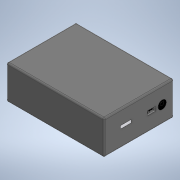
# Autodesk Inventor part: 22Ah BatteryPack
Saved by Autodesk Inventor 2021 (Build 250183000, 183)
## iProperties
Created: 2019-10-24
Part Number: 22Ah BatteryPack
Material: Generic
Document SubType Name: Modeling
Designer: jgray
Density: 1 g/cm^3
Appearance: Default
Author: jgray
Autodesk Inventor part; units mm, degrees
ref_plane "YZ Plane" through (0, 0, 0) normal (1, 0, 0) x (0, 1, 0)
ref_plane "XZ Plane" through (0, 0, 0) normal (0, 1, 0) x (-1, 0, 0)
ref_plane "XY Plane" through (0, 0, 0) normal (0, 0, 1) x (1, 0, 0)
sketch "Sketch1" plane through (0, 0, 0) normal (0, 1, 0) x (-1, 0, 0)
  line L0 (0, 0) -> (161, 0)
  line L1 (161, 0) -> (161, -115)
  line L2 (161, -115) -> (0, -115)
  line L3 (0, -115) -> (0, 0)
  dimension "d0" = 161
  dimension "d1" = 115
  constraints: 8 end point, 2 parallel, 1 horizontal, 1 perpendicular
  measures "d0" distance of L1.end L2.end
  measures "d1" distance of L0.end L1.end
extrude "Extrusion1" add sketch "Sketch1" along normal blind 56
fillet "Fillet1" radius 2.5 12 edges at (0, 56, -57.5) (0, 28, -115) (0, 28, 0) (0, 0, -57.5) (-80.5, 0, 0) (-80.5, 0, -115) (-80.5, 56, -115) (-80.5, 56, 0) (-161, 56, -57.5) (-161, 28, 0) (-161, 28, -115) (-161, 0, -57.5)
sketch "Sketch2" plane through (0, 2.5, -112.5) normal (1, 0, 0) x (0, 0, -1)
  line L0 (2.5, 0) -> (2.5, 51) projected
  line L1 (0, 0) -> (-110, 0) projected
  line L2 (0, 51) -> (0, 0) projected
  line L3 (-110, 51) -> (0, 51) projected
  line L4 (-110, 0) -> (-110, 51) projected
  line L5 (0, 53.5) -> (-110, 53.5) projected
  line L6 (-41.5, 29) -> (-27.5, 29)
  line L7 (-27.5, 29) -> (-27.5, 22)
  line L8 (-27.5, 22) -> (-41.5, 22)
  line L9 (-41.5, 22) -> (-41.5, 29)
  line L10 (-85, 30) -> (-67.5, 30)
  line L11 (-67.5, 30) -> (-67.5, 25)
  line L12 (-67.5, 25) -> (-85, 25)
  line L13 (-85, 25) -> (-85, 30)
  circle A0 centre (-30.5, 25.5) radius 2
  line L14 (-41.5, 22.5) -> (-35.5, 22.5)
  line L15 (-35.5, 22.5) -> (-35.5, 28.5)
  line L16 (-35.5, 28.5) -> (-41.5, 28.5)
  line L17 (-41.5, 28.5) -> (-41.5, 22.5)
  line L18 (-41.5, 22.5) -> (-35.5, 28.5) construction
  line L19 (-35.5, 22.5) -> (-41.5, 28.5) construction
  circle A1 centre (-16.5, 25.5) radius 7
  circle A2 centre (-16.5, 27.5) radius 3
  point P0 (-112.5, -2.5)
  point P1 (-38.5, 25.5)
  point P2 (-41.5, 22.5)
  dimension "d5" = 26
  dimension "d6" = 19
  dimension "d7" = 14
  dimension "d8" = 7
  dimension "d9" = 30
  dimension "d10" = 17.5
  dimension "d11" = 5
  dimension "d12" = 70
  dimension "d13" = 23.5
  dimension "d14" = 24.5
  dimension "d15" = 4
  dimension "d16" = 33
  dimension "d17" = 41
  dimension "d18" = 6
  dimension "d19" = 6
  dimension "d20" = 14
  dimension "d21" = 19
  dimension "d22" = 6
  dimension "d44" = 28
  dimension "d45" = 28
  dimension "d46" = 28
  constraints: 28 end point, 6 parallel, 3 centre point, 3 horizontal, 3 perpendicular, 2 coincident, 2 midpoint
  measures "d5" distance from line of L5 point (-16.5, 27.5)
  measures "d6" distance from line of L0 point (-16.5, 27.5)
  measures "d7" distance of L7.end L8.end
  measures "d8" distance of L6.end L7.end
  measures "d9" distance between parallel lines of L0 L7
  measures "d10" distance of L11.end L12.end
  measures "d11" distance of L10.end L11.end
  measures "d12" distance between parallel lines of L0 L11
  measures "d13" distance between parallel lines of L5 L10
  measures "d14" distance between parallel lines of L5 L6
  measures "d15" diameter of A0
  measures "d16" distance from line of L0 A0.centre
  measures "d17" distance from line of L0 point (-38.5, 25.5)
  measures "d18" distance of L16.end L15.end
  measures "d19" distance of L15.end L14.end
  measures "d20" diameter of A1
  measures "d21" distance from line of L0 A1.centre
  measures "d22" diameter of A2
  measures "d44" distance from line of A1.centre L5
  measures "d45" distance from line of L5 A0.centre
  measures "d46" distance from line of L5 point (-38.5, 25.5)
extrude "Extrusion2" cut sketch "Sketch2" against normal blind 10 contours A2
extrude "Extrusion3" cut sketch "Sketch2" against normal blind 0.1 contours A1
extrude "Extrusion4" cut sketch "Sketch2" against normal blind 10 contours A0
extrude "Extrusion5" cut sketch "Sketch2" against normal blind 5 contours L6 L7 L8 L9 L14 L15 L16 | L16 L15 L14 L9 | A0
extrude "Extrusion7" cut sketch "Sketch2" against normal blind 0.2 contours L10 L11 L12 L13
sketch "Sketch3" plane through (-10, 30, -96) normal (1, 0, 0) x (0, 0, -1)
  circle A0 centre (0, 0) radius 1.25
  point P0 (-96, -30)
  dimension "d35" = 2.5
  constraints: 1 centre point
  measures "d35" diameter of A0
extrude "Extrusion8" add sketch "Sketch3" along normal blind 8
fillet "Fillet2" radius 1.25 1 edges at (-2, 30, -94.75)
sketch "Sketch4" plane through (-5, 2.5, -112.5) normal (1, 0, 0) x (0, 0, -1)
  circle A0 centre (-38.5, 25.5) radius 1.4
  circle A1 centre (-38.5, 25.5) radius 0.9
  point P0 (-112.5, -2.5)
  dimension "d39" = 2.8
  dimension "d40" = 1.8
  constraints: 2 centre point, 2 coincident
  measures "d39" diameter of A0
  measures "d40" diameter of A1
extrude "Extrusion9" add sketch "Sketch4" along normal blind 5
fillet "Fillet3" radius 0.25 2 edges at (0, 28, -73.1) (0, 28, -72.6)
body "Solid1"
